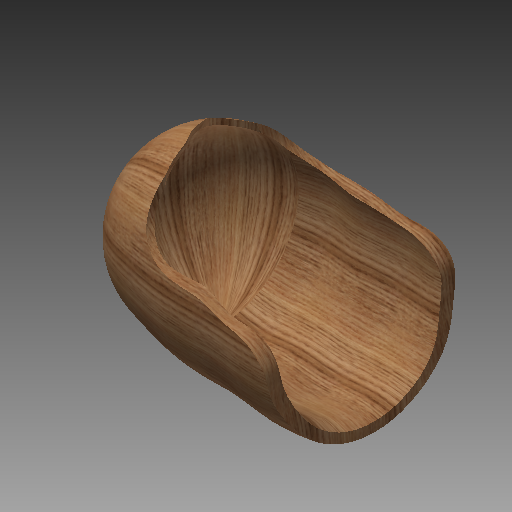
# Autodesk Inventor part: 3D HUMAN
Saved by Autodesk Inventor 2022 (Build 260153000, 153)
## iProperties
Category: PART
Part Number: 3D HUMAN
Document SubType Name: Modeling
Created: 2003-07-26
Designer: M.F.
Manufacturer: Standard
Standards Organization: Custom
Catalog Web Link: www.apollocanard.com
Density: 1 g/cm^3
Material: Generic
Appearance: Wood (Oak)
Control State: 0
Master: False
Checked Out: False
Shininess: 64.0
Length Units: 11272
Angle Units: 11279
Time Units: 11290
Mass Units: 11286
Length Display Precision: 3
Angle Display Precision: 2
Compacted: True
Density: 0.0
Volumn: 0.0
Area: 0.0
PropertySet Name: Model Information
Title: iMandy
Author: M.F.
Autodesk Inventor part; units mm, degrees
ref_plane "YZ Plane" through (0, 0, 0) normal (1, 0, 0) x (0, 1, 0)
ref_plane "XZ Plane" through (0, 0, 0) normal (0, 1, 0) x (-1, 0, 0)
ref_plane "XY Plane" through (0, 0, 0) normal (0, 0, 1) x (1, 0, 0)
sketch "Sketch2" plane through (0, 0, 0) normal (1, 0, 0) x (0, 1, 0)
  line L0 (98.6956, 0) -> (92.3456, 0)
  arc A0 (0, -92.3456) -> (92.3456, 0) centre (0, 0) ccw
  line L1 (0, 0) -> (0, -92.3456) construction
  line L2 (0, 0) -> (92.3456, 0) construction
  spline S0 degree 3 poles (98.6956, 0) (98.3274, -6.4013) (97.467, -21.3587) (89.1602, -45.1554) (71.8286, -70.2021) (45.9972, -89.8913) (11.2541, -98.5005) (-21.5615, -106.6242) (-56.7983, -109.8163) (-91.3614, -107.5862) (-128.4576, -112.4433) (-156.1625, -113.7837) (-205.1871, -107.936) (-166.6438, -94.2729) (-141.4099, -96.6139) (-105.953, -100.7479) (-68.096, -91.0455) (-32.2758, -101.1707) (-10.3133, -95.1656) (0, -92.3456) knots 0 0 0 0 1.918173 4.482082 7.437092 10.970107 13.921257 18.07952 21.136871 24.450103 28.588923 31.67221 34.69416 37.117519 39.287936 43.295456 47.296513 50.862903 54.020344 54.020344 54.020344 54.020344
  arc A1 (15.24, -97.5119) -> (98.6956, 0) centre (0, 0) ccw construction
  line L3 (0, -92.3456) -> (-190.5, -105.6667) construction
  point P0 (0, 0)
  point P1 (0, 0)
  point P2 (96.8316, -19.091)
  point P3 (88.6468, -43.3885)
  point P4 (71.8291, -67.6861)
  point P5 (43.3885, -88.6468)
  point P6 (-25.4, -106.3156)
  point P7 (-55.857, -108.9825)
  point P8 (-88.9885, -108.7531)
  point P9 (-130.2373, -112.1468)
  point P10 (-106.3571, -98.2551)
  point P11 (-66.5277, -94.4515)
  point P12 (-31.0491, -98.0815)
  point P13 (-146.3804, -96.216)
  point P14 (-161.0679, -112.5203)
  point P15 (-168.0832, -96.4605)
  dimension "d40" = 92.3456
  dimension "d47" = 190.5
  dimension "d51" = 15.24
  dimension "d52" = 6.35
  dimension "d54" = 13.97
  dimension "d55" = 4
  dimension "d56" = 7.62
  dimension "d57" = 6.35
  dimension "d58" = 1.524
  dimension "d59" = 2.54
  dimension "d60" = 3.556
  dimension "d61" = 8.89
  dimension "d62" = 10.668
  dimension "d63" = 10.16
  dimension "d64" = 12.7
  constraints: 8 end point, 8 point on circle, 2 centre point, 2 coincident, 2 perpendicular, 1 horizontal, 1 point on line, 19 other
  measures "d40" radius of A0
  measures "d47" distance from line of L3.end L1
  measures "d51" distance from line of A1.start L1
  measures "d52" distance of L0.start L0.end
  measures "d54" vertical distance of point (-25.4, -106.316) L1.end
  measures "d55" angle of L3 L2
  measures "d56" distance from line of L3 point (-168.083, -96.461)
  measures "d57" distance from line of point (-146.38, -96.216) L3
  measures "d58" distance from line of point (-106.357, -98.255) L3
  measures "d59" distance from line of point (-66.528, -94.452) L3
  measures "d60" distance from line of L3 point (-31.049, -98.081)
  measures "d61" distance from line of point (-161.068, -112.52) L3
  measures "d62" distance from line of L3 point (-130.237, -112.147)
  measures "d63" distance from line of point (-88.988, -108.753) L3
  measures "d64" distance from line of point (-55.857, -108.983) L3
revolve "Revolution2" add sketch "Sketch2" angle 360 about axis through (0, 0, 0) along (0, 1, 0)
sketch "Sketch8" plane through (0, 0, 0) normal (1, 0, 0) x (0, 1, 0)
  line L0 (10.16, 139.7) -> (-198.12, 139.7)
  line L1 (-198.12, 139.7) -> (-198.12, -139.7)
  spline S0 degree 3 poles (10.16, 139.7) (11.9904, 130.1887) (16.1915, 108.3589) (12.0398, 77.6704) (2.6421, 48.7789) (-21.0997, 32.7678) (-49.9835, 28.5214) (-80.4221, 29.3394) (-109.7065, 18.4501) (-140.5214, 21.1518) (-167.0503, -1.1524) (-166.236, -32.7088) (-177.8445, -62.0804) (-180.9235, -94.7923) (-182.4881, -124.6077) (-194.6728, -136.3718) (-198.12, -139.7) knots 0 0 0 0 2.887156 6.626461 9.223954 11.677489 14.724368 17.883389 20.731029 23.938935 26.839851 29.804674 32.924718 36.216502 39.791985 41.202612 41.202612 41.202612 41.202612
  line L2 (10.16, 139.7) -> (10.16, 73.9604) construction
  point P0 (0, 0)
  point P1 (0, 0)
  point P2 (14.2875, 111.125)
  point P3 (-19.8019, 35.5682)
  point P4 (-81.1633, 27.2541)
  point P5 (-108.913, 20.8623)
  point P6 (-140.7071, 16.5954)
  point P7 (0, 50.055)
  point P8 (-49.6491, 29.4451)
  point P9 (-162.5389, -2.507)
  point P10 (-168.1694, -31.6156)
  point P11 (-176.2203, -61.7595)
  point P12 (-180.6478, -94.3782)
  point P13 (-188.6782, -129.2195)
  dimension "d45" = 139.7
  dimension "d49" = 139.7
  dimension "d65" = 10.16
  dimension "d66" = 208.28
  constraints: 6 end point, 1 coincident, 1 horizontal, 1 parallel, 1 perpendicular, 16 other
  measures "d45" distance from line of L0 point (0, 0)
  measures "d49" vertical distance of L1.end point (0, 0)
  measures "d65" horizontal distance of L0.start point (0, 0)
  measures "d66" distance of L0.start L0.end
extrude "Extrusion3" cut sketch "Sketch8" along normal through all both and the other way through all
sketch "Sketch9" plane through (0, 0, 0) normal (0, 0, 1) x (1, 0, 0)
  arc A0 (33.2444, 47.257) -> (63.9166, 5.9223) centre (88.4127, 56.147) ccw
  line L0 (52.3562, -17.78) -> (-63.5, -17.78)
  spline S0 degree 3 poles (33.2444, 47.257) (27.5944, 43.8889) (16.5976, 37.3337) (-2.5379, 32.8216) (-17.8963, 21.032) (-36.8804, 17.7503) (-53.2606, 12.8563) (-68.6707, 0.3135) (-65.2943, -11.5014) (-63.5, -17.78) knots 0 0 0 0 1.963535 3.821656 5.810787 7.620816 9.478937 11.053291 12.838721 12.838721 12.838721 12.838721
  line L1 (63.9166, 5.9223) -> (52.3562, -17.78)
  point P0 (0, 0)
  point P1 (0, 0)
  point P2 (15.875, 38.1)
  point P3 (-1.5875, 31.75)
  point P4 (-19.05, 22.225)
  point P5 (-36.5125, 17.4625)
  point P6 (-53.975, 11.1125)
  point P7 (-65.1272, 0)
  dimension "d67" = 17.78
  dimension "d68" = 33.2444
  dimension "d70" = 55.88
  dimension "d80" = 47.257
  dimension "d87" = 8.89
  dimension "d89" = 63.5
  dimension "d90" = 64
  constraints: 4 end point, 2 point on circle, 1 centre point, 1 coincident, 1 horizontal, 1 point on line, 9 other
  measures "d67" distance from line of L0 point (0, 0)
  measures "d68" horizontal distance of A0.start point (0, 0)
  measures "d70" radius of A0
  measures "d80" vertical distance of A0.start point (0, 0)
  measures "d87" vertical distance of A0.centre A0.start
  measures "d89" horizontal distance of L0.end point (0, 0)
  measures "d90" angle of L0 L1
extrude "Extrusion5" cut sketch "Sketch9" along normal through all
body "Solid2"
